Autodesk Inventor part; units mm, degrees
(part 3 of 3)
sketch "Sketch21" plane through (0, 5.08, 0) normal (0, 1, 0) x (1, 0, 0)
  circle A0 centre (93.5166, 87.7325) radius 2.5067
  circle A1 centre (43.4064, 87.8565) radius 2.5067
  circle A2 centre (43.4064, 137.8857) radius 2.5067
  circle A3 centre (93.4273, 137.9376) radius 2.5067
  circle A4 centre (68.4419, 113.0884) radius 29.9448
  line L0 (68.4419, 83.1436) -> (68.4419, 143.0333)
  line L1 (62.7753, 83.6846) -> (62.7753, 142.4922)
  line L2 (74.1086, 83.6846) -> (74.1086, 142.4922)
  line L3 (57.1609, 85.3498) -> (57.1609, 140.827)
  line L4 (50.6919, 88.9714) -> (50.6919, 137.2055)
  line L5 (44.4794, 95.1304) -> (44.4794, 131.0464)
  line L6 (79.723, 85.3498) -> (79.723, 140.827)
  line L7 (86.1919, 88.9714) -> (86.1919, 137.2055)
  line L8 (92.4045, 95.1304) -> (92.4045, 131.0464)
  line L9 (98.3868, 113.0884) -> (38.4971, 113.0884)
  line L10 (39.2589, 106.3767) -> (97.6249, 106.3767)
  line L11 (39.2589, 119.8001) -> (97.6249, 119.8001)
  line L12 (41.9244, 126.9993) -> (94.9595, 126.9993)
  line L13 (46.4105, 133.3692) -> (90.4734, 133.3692)
  line L14 (53.778, 139.1971) -> (83.1058, 139.1971)
  line L15 (94.9595, 99.1776) -> (41.9244, 99.1776)
  line L16 (46.4105, 92.8077) -> (90.4734, 92.8077)
  line L17 (82.3359, 86.562) -> (54.5479, 86.562)
  point P0 (0, 0)
  constraints: 36 end point, 15 parallel, 4 centre point, 1 horizontal, 1 perpendicular, 1 vertical, 38 other
extrude "Extrusion19" cut sketch "Sketch21" against normal blind 6.35 contours A0 | A1 | A2 | A3 | L9 L8 L11 A4 | A4 L10 L8 L9 | L11 L8 L12 A4 | A4 L15 L8 L10 | L12 L8 A4 | A4 L8 L15 | L9 L6 L11 L7 | L7 L10 L6 L9 | L11 L6 L12 L7 | L7 L15 L6 L10 | L12 L6 L13 L7 | L7 L16 L6 L15 | L9 L0 L11 L2 | L2 L10 L0 L9 | L7 L13 L6 L14 A4 | L11 L0 L12 L2 | A4 L17 L6 L16 L7 | L2 L15 L0 L10 | L9 L1 L11 L0 | L0 L10 L1 L9 | L14 L6 A4 | L12 L0 L13 L2 | L11 L1 L12 L0 | A4 L6 L17 | L2 L16 L0 L15 | L0 L15 L1 L10 | L13 L0 L14 L2 | L12 L1 L13 L0 | L2 L17 L0 L16 | L0 L16 L1 L15 | L9 L4 L11 L3 | L3 L10 L4 L9 | L2 L14 L0 A4 | L13 L1 L14 L0 | L11 L4 L12 L3 | A4 L0 L17 L2 | L0 L17 L1 L16 | L3 L15 L4 L10 | L0 L14 L1 A4 | L12 L4 L13 L3 | A4 L1 L17 L0 | L3 L16 L4 L15 | L9 A4 L11 L5 | L5 L10 A4 L9 | L13 L4 A4 L14 L3 | L11 A4 L12 L5 | L3 L17 A4 L4 L16 | L5 L15 A4 L10 | L3 L14 A4 | L12 A4 L5 | A4 L17 L3 | L5 A4 L15
fillet "Fillet1" radius 3.175 12 edges at (-117.475, 43.18, -134.9375) (-117.475, 43.18, -107.95) (-117.475, 43.18, -80.9625) (-117.475, 43.18, -58.7375) (-117.475, 43.18, -31.75) (-117.475, 43.18, -4.7625) (-117.475, 43.18, 17.4625) (-117.475, 43.18, 44.45) (-117.475, 43.18, 71.4375) (-117.475, 43.18, 93.6625) (-117.475, 43.18, 120.65) (-117.475, 43.18, 147.6375)
equation "\"d80\" = d78"
equation "\"d84\" = d78"
equation "\"d89\" = d78"
equation "\"d101\" = d78"
equation "\"BendRadius\" = Thickness"
equation "\"BendReliefWidth\" = Thickness"
equation "\"BendReliefDepth\" = 0.5 * Thickness"
equation "\"CornerReliefSize\" = 4 * Thickness"
equation "\"MinimumRemnant\" = 2 * Thickness"
equation "\"TransitionRadius\" = BendRadius"
equation "\"JacobiRadiusSize\" = BendRadius"
equation "\"GapSize\" = Thickness"
equation "\"Thickness\" = 3.048"
body "Solid1"
